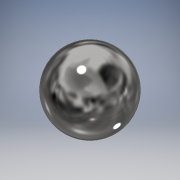
# Autodesk Inventor part: BEaring 608 Ball Bearing
Saved by Autodesk Inventor 2018 (Build 220112000, 112)
## iProperties
Created: 2017-09-15
Part Number: BEaring 608 Ball Bearing
Material: Steel, Alloy
Document SubType Name: Modeling
Designer: Rus
Density: 7.73 g/cm^3
Appearance: Steel - Polished
Author: Rus
Autodesk Inventor part; units mm, degrees
ref_plane "YZ Plane" through (0, 0, 0) normal (1, 0, 0) x (0, 1, 0)
ref_plane "XZ Plane" through (0, 0, 0) normal (0, 1, 0) x (-1, 0, 0)
ref_plane "XY Plane" through (0, 0, 0) normal (0, 0, 1) x (1, 0, 0)
sketch "Sketch1" plane through (0, 0, 0) normal (0, 0, 1) x (1, 0, 0)
  circle A0 centre (0, 0) radius 1.9844
  line L0 (0, 0) -> (0, -1.9844)
  line L1 (0, 0) -> (0, 1.9844)
  dimension "d0" = 3.9688
  constraints: 4 end point, 2 point on circle, 1 centre point, 1 coincident, 1 point on line, 1 vertical
  measures "d0" diameter of A0
revolve "Revolution1" add sketch "Sketch1" angle 360 about axis through (0, 0, 0) along (0, 1, 0) picked at (-0.1583, -1.3037) contours L1 L0 A0
body "Solid1"
